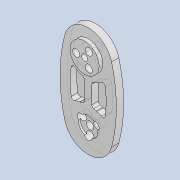
# Autodesk Inventor part: 原動節1-3
Saved by Autodesk Inventor 2020 (Build 240168000, 168)
## iProperties
Created: 2020-10-27
Part Number: 原動節1-3
Material: アルミニウム 2014-T4
Document SubType Name: Modeling
Designer: AA19065
Density: 2.8 g/cm^3
Appearance: サテン
Mass: 6.36426 g
Surface Area: 21.4383 cm^2
Volume: 2.27295 cm^3
Author: AA19065
Autodesk Inventor part; units mm, degrees
ref_plane "YZ Plane" through (0, 0, 0) normal (1, 0, 0) x (0, 1, 0)
ref_plane "XZ Plane" through (0, 0, 0) normal (0, 1, 0) x (-1, 0, 0)
ref_plane "XY Plane" through (0, 0, 0) normal (0, 0, 1) x (1, 0, 0)
sketch "スケッチ1" plane through (0, 0, 0) normal (0, 0, 1) x (1, 0, 0)
  circle A0 centre (-9.6968, -10.9779) radius 1.5
  circle A1 centre (-15.759, -10.9779) radius 1.5
  circle A2 centre (-12.7279, -12.7279) radius 1.25
  circle A3 centre (-12.7279, -16.2279) radius 1.5
  circle A4 centre (-12.7279, -12.7279) radius 6
  line L0 (-12.7279, -12.7279) -> (-12.7279, 12.7279) construction
  circle A5 centre (-12.7279, 12.7279) radius 1.25
  circle A6 centre (-16.2279, 12.7279) radius 1.5
  circle A7 centre (-10.9779, 9.6968) radius 1.5
  circle A8 centre (-10.9779, 15.759) radius 1.5
  circle A9 centre (-12.7279, 12.7279) radius 6
  arc A10 (-18.1192, 15.3613) -> (-18.1192, -15.3613) centre (13.3297, 0) ccw
  arc A11 (-7.3367, -15.3613) -> (-7.3367, 15.3613) centre (-38.7856, 0) ccw
  circle A12 centre (-12.7279, -12.7279) radius 1.5
  line L1 (-16.2279, 12.7279) -> (-12.7279, 12.7279) construction
  point P0 (0, 0)
  point P1 (0, 0)
  dimension "d2" = 360
  dimension "d3" = 3.5
  dimension "d4" = 35
  dimension "d5" = 3
  dimension "d22" = 2.5
  constraints: 13 centre point, 8 point on circle, 7 equal radius, 4 end point, 4 tangent, 3 coincident, 1 perpendicular, 1 vertical, 10 other
  measures "d3" distance of A5.centre L1.start
  measures "d4" radius of A11
  measures "d5" diameter of A12
  measures "d22" diameter of A2
extrude "押し出し1" add sketch "スケッチ1" along normal blind 3 contours A4 | A4 A10 A9 A11 | A9
extrude "押し出し2" add sketch "スケッチ1" along normal blind 0.3 contours A6 | A7 | A8
sketch "スケッチ2" plane through (0, 0, 3) normal (0, 0, 1) x (1, 0, 0)
  circle A0 centre (-12.7279, -12.7279) radius 1.5 projected
  circle A1 centre (-12.7279, -12.7279) radius 4
  point P0 (0, 0)
  dimension "d11" = 8
  constraints: 1 centre point, 1 coincident
  measures "d11" diameter of A1
extrude "押し出し3" cut sketch "スケッチ2" against normal blind 0.8 contours A0 | A1
sketch "スケッチ3" plane through (0, 0, 3) normal (0, 0, 1) x (1, 0, 0)
  arc A0 (-16.6869, -12.1565) -> (-14.2125, -16.4422) centre (-12.7279, -12.7279) ccw projected
  arc A1 (-15.2023, -9.5851) -> (-16.6869, -12.1565) centre (-15.759, -10.9779) ccw projected
  arc A2 (-10.2536, -9.5851) -> (-15.2023, -9.5851) centre (-12.7279, -12.7279) ccw projected
  arc A3 (-8.7689, -12.1565) -> (-10.2536, -9.5851) centre (-9.6968, -10.9779) ccw projected
  arc A4 (-11.2433, -16.4422) -> (-8.7689, -12.1565) centre (-12.7279, -12.7279) ccw projected
  arc A5 (-14.2125, -16.4422) -> (-11.2433, -16.4422) centre (-12.7279, -16.2279) ccw projected
  circle A6 centre (-10.9779, 9.6968) radius 1.5 projected
  circle A7 centre (-12.7279, 12.7279) radius 1.25 projected
  circle A8 centre (-16.2279, 12.7279) radius 1.5 projected
  circle A9 centre (-10.9779, 15.759) radius 1.5 projected
  arc A10 (-7.3367, 15.3613) -> (-18.1192, 15.3613) centre (-12.7279, 12.7279) ccw projected
  arc A11 (-18.1192, 15.3613) -> (-18.1192, -15.3613) centre (13.3297, 0) ccw projected
  arc A12 (-18.1192, -15.3613) -> (-7.3367, -15.3613) centre (-12.7279, -12.7279) ccw projected
  arc A13 (-7.3367, -15.3613) -> (-7.3367, 15.3613) centre (-38.7856, 0) ccw projected
  circle A14 centre (-12.7279, 12.7279) radius 6
  point P0 (0, 0)
  point P1 (-18.1192, 15.3613)
  point P2 (-7.3367, 15.3613)
  dimension "d14" = 12
  constraints: 1 centre point, 1 coincident
  measures "d14" diameter of A14
extrude "押し出し4" add sketch "スケッチ3" along normal blind 1.5 contours A14 A10
sketch "スケッチ4" plane through (0, 0, 0) normal (0, 0, -1) x (-1, 0, 0)
  arc A0 (7.3367, 15.3613) -> (18.1192, 15.3613) centre (12.7279, 12.7279) ccw projected
  arc A1 (7.3367, 15.3613) -> (7.3367, -15.3613) centre (38.7856, 0) ccw projected
  arc A2 (7.3367, -15.3613) -> (18.1192, -15.3613) centre (12.7279, -12.7279) ccw projected
  arc A3 (18.1192, -15.3613) -> (18.1192, 15.3613) centre (-13.3297, 0) ccw projected
  arc A4 (18.1192, 15.3613) -> (7.3367, 15.3613) centre (12.7279, 12.7279) ccw projected
  circle A5 centre (12.7279, 12.7279) radius 1.25 projected
  circle A6 centre (9.6968, -10.9779) radius 1.5 projected
  circle A7 centre (12.7279, -16.2279) radius 1.5 projected
  circle A8 centre (15.759, -10.9779) radius 1.5 projected
  circle A9 centre (12.7279, -12.7279) radius 1.5 projected
  circle A10 centre (12.7279, 12.7279) radius 10
  circle A11 centre (12.7279, -12.7279) radius 10
  point P0 (0, 0)
  point P1 (4.5014, -7.0425)
  point P2 (20.9545, -7.0425)
  point P3 (20.9545, 7.0425)
  point P4 (4.5014, 7.0425)
  dimension "d17" = 20
  dimension "d18" = 20
  constraints: 2 centre point, 2 coincident
  measures "d17" diameter of A10
  measures "d18" diameter of A11
extrude "押し出し5" add sketch "スケッチ4" against normal up to surface (3 mm away) contours A1 A10 A3 A4 | A1 A2 A3 A11 picked at (19.9443, -14.4106)
fillet "フィレット1" radius 2 4 edges at (-4.5014, -7.0425, 1.5) (-20.9545, -7.0425, 1.5) (-20.9545, 7.0425, 1.5) (-4.5014, 7.0425, 1.5)
sketch "スケッチ5" plane through (0, 0, 3) normal (0, 0, 1) x (1, 0, 0)
  circle A0 centre (-12.7279, 12.7279) radius 6 projected
  arc A1 (-21.1019, 6.2819) -> (-21.1019, -6.2819) centre (13.3297, 0) ccw projected
  arc A2 (-21.3459, -7.6554) -> (-21.1019, -6.2819) centre (-23.0695, -6.6408) ccw projected
  arc A3 (-21.3459, -7.6554) -> (-4.11, -7.6554) centre (-12.7279, -12.7279) ccw projected
  arc A4 (-4.3539, -6.2819) -> (-4.11, -7.6554) centre (-2.3864, -6.6408) ccw projected
  arc A5 (-4.3539, -6.2819) -> (-4.3539, 6.2819) centre (-38.7856, 0) ccw projected
  arc A6 (-4.11, 7.6554) -> (-4.3539, 6.2819) centre (-2.3864, 6.6408) ccw projected
  arc A7 (-4.11, 7.6554) -> (-21.3459, 7.6554) centre (-12.7279, 12.7279) ccw projected
  arc A8 (-21.1019, 6.2819) -> (-21.3459, 7.6554) centre (-23.0695, 6.6408) ccw projected
  arc A9 (-16.6869, -12.1565) -> (-14.2125, -16.4422) centre (-12.7279, -12.7279) ccw projected
  arc A10 (-15.2023, -9.5851) -> (-16.6869, -12.1565) centre (-15.759, -10.9779) ccw projected
  arc A11 (-10.2536, -9.5851) -> (-15.2023, -9.5851) centre (-12.7279, -12.7279) ccw projected
  arc A12 (-8.7689, -12.1565) -> (-10.2536, -9.5851) centre (-9.6968, -10.9779) ccw projected
  arc A13 (-11.2433, -16.4422) -> (-8.7689, -12.1565) centre (-12.7279, -12.7279) ccw projected
  arc A14 (-14.2125, -16.4422) -> (-11.2433, -16.4422) centre (-12.7279, -16.2279) ccw projected
  arc A15 (-19.6263, 6.0126) -> (-19.6263, -6.0126) centre (13.3297, 0) ccw
  arc A16 (-19.6263, 6.0126) -> (-20.0532, 8.4162) centre (-23.0695, 6.6408) ccw
  arc A17 (-5.4027, 8.4162) -> (-20.0532, 8.4162) centre (-12.7279, 12.7279) ccw
  arc A18 (-5.4027, 8.4162) -> (-5.8295, 6.0126) centre (-2.3864, 6.6408) ccw
  arc A19 (-5.8295, -6.0126) -> (-5.8295, 6.0126) centre (-38.7856, 0) ccw
  arc A20 (-5.8295, -6.0126) -> (-5.4027, -8.4162) centre (-2.3864, -6.6408) ccw
  arc A21 (-20.0532, -8.4162) -> (-5.4027, -8.4162) centre (-12.7279, -12.7279) ccw
  arc A22 (-20.0532, -8.4162) -> (-19.6263, -6.0126) centre (-23.0695, -6.6408) ccw
  circle A23 centre (-12.7279, 12.7279) radius 8.8048
  arc A24 (-16.1038, -5.6216) -> (-20.5701, -13.3575) centre (-15.759, -10.9779) ccw
  arc A25 (-20.5701, -13.3575) -> (-17.1943, -19.2047) centre (-12.7279, -12.7279) ccw
  arc A26 (-17.1943, -19.2047) -> (-8.2616, -19.2047) centre (-12.7279, -16.2279) ccw
  arc A27 (-8.2616, -19.2047) -> (-4.8857, -13.3575) centre (-12.7279, -12.7279) ccw
  arc A28 (-4.8857, -13.3575) -> (-9.3521, -5.6216) centre (-9.6968, -10.9779) ccw
  arc A29 (-9.3521, -5.6216) -> (-16.1038, -5.6216) centre (-12.7279, -12.7279) ccw
  line L0 (-12.7279, 12.7279) -> (-12.7279, -12.7279)
  line L1 (-14.2279, 12.7279) -> (-14.2279, -12.7279)
  line L2 (-11.2279, 12.7279) -> (-11.2279, -12.7279)
  point P0 (0, 0)
  point P1 (-19.6234, 7.2529)
  point P2 (-19.6234, -7.2529)
  point P3 (-5.8325, 7.2529)
  point P4 (-11.2279, 4.0519)
  point P5 (-11.2279, -5.0048)
  point P6 (-5.8325, -7.2529)
  point P7 (-14.2279, -5.0048)
  point P8 (-14.2279, 4.0519)
  dimension "d23" = 1.5
  dimension "d24" = 1.5
  dimension "d25" = 1.5
  constraints: 31 point on circle, 14 centre point, 6 end point, 2 parallel, 1 vertical, 15 other
  measures "d23" radial gap between concentric circles of A1 A15
  measures "d24" distance between parallel lines of L0 L1
  measures "d25" distance between parallel lines of L0 L2
extrude "押し出し6" cut sketch "スケッチ5" against normal blind 2.7 contours L1 A29 A24 A22 A15 A16 A23 | A23 A18 A19 A20 A28 A29 L2
fillet "フィレット2" radius 1.05 10 edges at (-19.6234, 7.2529, 1.65) (-5.8325, 7.2529, 1.65) (-11.2279, 4.0519, 1.65) (-14.2279, 4.0519, 1.65) (-19.6234, -7.2529, 1.65) (-14.2279, -5.0048, 1.65) (-11.2279, -5.0048, 1.65) (-5.8325, -7.2529, 1.65) (-9.3521, -5.6216, 1.65) (-16.1038, -5.6216, 1.65)
sketch "スケッチ6" plane through (0, 0, 0) normal (0, 0, -1) x (-1, 0, 0)
  arc A0 (21.3459, 7.6554) -> (4.11, 7.6554) centre (12.7279, 12.7279) ccw projected
  arc A1 (4.3539, 6.2819) -> (4.11, 7.6554) centre (2.3864, 6.6408) ccw projected
  arc A2 (4.3539, 6.2819) -> (4.3539, -6.2819) centre (38.7856, 0) ccw projected
  arc A3 (4.11, -7.6554) -> (4.3539, -6.2819) centre (2.3864, -6.6408) ccw projected
  arc A4 (4.11, -7.6554) -> (21.3459, -7.6554) centre (12.7279, -12.7279) ccw projected
  arc A5 (21.1019, -6.2819) -> (21.3459, -7.6554) centre (23.0695, -6.6408) ccw projected
  arc A6 (21.1019, -6.2819) -> (21.1019, 6.2819) centre (-13.3297, 0) ccw projected
  arc A7 (21.3459, 7.6554) -> (21.1019, 6.2819) centre (23.0695, 6.6408) ccw projected
  circle A8 centre (12.7279, 12.7279) radius 1.25 projected
  circle A9 centre (9.6968, -10.9779) radius 1.5 projected
  circle A10 centre (12.7279, -16.2279) radius 1.5 projected
  circle A11 centre (15.759, -10.9779) radius 1.5 projected
  circle A12 centre (12.7279, -12.7279) radius 1.5 projected
  arc A13 (3.0573, 15.2735) -> (3.0573, -15.2735) centre (61.0808, 0) ccw
  arc A14 (22.3985, -15.2735) -> (22.3985, 15.2735) centre (-35.6249, 0) ccw
  arc A15 (21.3459, 7.6554) -> (4.11, 7.6554) centre (12.7279, 12.7279) ccw projected
  arc A16 (4.11, -7.6554) -> (21.3459, -7.6554) centre (12.7279, -12.7279) ccw projected
  point P0 (0, 0)
  dimension "d29" = 60
  constraints: 8 point on circle, 4 tangent, 2 centre point, 1 equal radius
  measures "d29" radius of A14
extrude "押し出し7" add sketch "スケッチ6" against normal up to surface (3 mm away) contours A0 A14 A4 A5 A6 A7 | A0 A1 A2 A3 A4 A13
equation "\"d3\" = d6"
equation "\"d6\" = 3.5"
